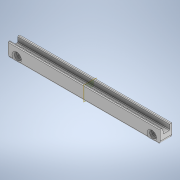
# Autodesk Inventor part: DisplayHolderLower
Saved by Autodesk Inventor 2022 (Build 260153000, 153)
## iProperties
Created: 2021-04-23
Part Number: DisplayHolderLower
Material: Generic
Document SubType Name: Modeling
Designer: Viktor
Density: 1 g/cm^3
Appearance: Default
Author: Viktor
## iProperties of the stored document DisplayHolderLower_3DPrint.ipt
Created: 2021-04-23
Part Number: DisplayHolderLower_3DPrint
Material: Generic
Document SubType Name: Modeling
Designer: Viktor
Density: 1 g/cm^3
Appearance: Default
Author: Viktor
Autodesk Inventor part; units mm, degrees
ref_plane "YZ Plane" through (0, 0, 0) normal (1, 0, 0) x (0, 1, 0)
ref_plane "XZ Plane" through (0, 0, 0) normal (0, 1, 0) x (-1, 0, 0)
ref_plane "XY Plane" through (0, 0, 0) normal (0, 0, 1) x (1, 0, 0)
sketch "Sketch1" plane through (0, 0, 0) normal (0, 0, 1) x (1, 0, 0)
  line L0 (-12.5, -10) -> (12.5, -10)
  line L1 (12.5, -10) -> (12.5, 10)
  line L2 (12.5, 10) -> (-12.5, 10)
  line L3 (-12.5, 10) -> (-12.5, -10)
  line L4 (-12.5, -10) -> (12.5, 10) construction
  line L5 (12.5, -10) -> (-12.5, 10) construction
  point P0 (0, 0)
  dimension "d0" = 25
  dimension "d1" = 20
  constraints: 12 end point, 2 midpoint, 2 parallel, 1 horizontal, 1 perpendicular
  measures "d0" distance of L1.end L2.end
  measures "d1" distance of L0.end L1.end
extrude "Extrusion1" add sketch "Sketch1" along normal blind 17
sketch "Sketch2" plane through (-12.5, 10, 0) normal (0, 1, 0) x (1, 0, 0)
  line L0 (0, 0) -> (0, -17) projected
  line L1 (25, 0) -> (25, -17) projected
  line L2 (0, -2.8) -> (25, -2.8)
  line L3 (25, -2.8) -> (25, -12.4)
  line L4 (25, -12.4) -> (0, -12.4)
  line L5 (0, -12.4) -> (0, -2.8)
  line L6 (25, 0) -> (0, 0) projected
  point P0 (12.5, 0)
  point P1 (0, -12.4)
  dimension "d4" = 2.8
  dimension "d5" = 9.6
  constraints: 8 end point, 2 parallel, 2 point on line, 1 horizontal, 1 perpendicular
  measures "d4" distance between parallel lines of L6 L2
  measures "d5" distance between parallel lines of L4 L2
extrude "Extrusion2" cut sketch "Sketch2" against normal blind 8 contours L2 L1 L4 L0
chamfer "Chamfer1" distance 2 angle 70 1 edges at (0, 10, 12.4) measured on face at (0, 10, 12.9)
fillet "Fillet1" radius 1 5 edges at (0, 2, 12.4) (0, 2, 2.8) (0, 10, 14.4) (0, 10, 17) (0, 10, 2.8)
sketch "Sketch3" plane through (0, 0, 17) normal (0, 0, 1) x (1, 0, 0)
  line L0 (0, 14) -> (0, -14) projected
  circle A0 centre (0, -4) radius 2.4
  line L1 (-12.5, -10) -> (12.5, -10) projected
  point P0 (0, 0)
  dimension "d12" = 4.8
  dimension "d13" = 6
  constraints: 1 centre point, 1 point on line
  measures "d12" diameter of A0
  measures "d13" distance from line of L1 A0.centre
extrude "Extrusion3" cut sketch "Sketch3" against normal through all
sketch "Sketch4" plane through (0, 0, 17) normal (0, 0, 1) x (1, 0, 0)
  circle A0 centre (0, -4) radius 2.4 projected
  circle A1 centre (0, -4) radius 5
  point P0 (0, 0)
  dimension "d16" = 10
  constraints: 1 centre point, 1 coincident
  measures "d16" diameter of A1
extrude "Extrusion4" cut sketch "Sketch4" against normal blind 5 contours A0 | A1
chamfer "Chamfer2" distance 2 angle 45 1 edges at (-5, -4, 17)
sketch "Sketch6" plane through (-12.5, -10, 0) normal (-1, 0, 0) x (0, 0, 1)
  arc A0 (2.8, 19) -> (1.8, 20) centre (1.8, 19) ccw projected
  line L0 (0, 20) -> (1.8, 20) projected
  line L1 (0, 20) -> (0, 0) projected
  line L2 (0, 0) -> (17, 0) projected
  line L3 (17, 19) -> (17, 0) projected
  arc A1 (17, 19) -> (16, 20) centre (16, 19) ccw projected
  line L4 (15.1002, 20) -> (16, 20) projected
  arc A2 (15.1002, 20) -> (14.1605, 19.342) centre (15.1002, 19) ccw projected
  line L5 (12.4, 14.505) -> (14.1605, 19.342) projected
  line L6 (12.4, 14.505) -> (12.4, 13) projected
  arc A3 (11.4, 12) -> (12.4, 13) centre (11.4, 13) ccw projected
  line L7 (11.4, 12) -> (3.8, 12) projected
  arc A4 (2.8, 13) -> (3.8, 12) centre (3.8, 13) ccw projected
  line L8 (2.8, 13) -> (2.8, 19) projected
  point P0 (0, 10)
extrude "Extrusion6" add sketch "Sketch6" along normal blind 87.5
ref_plane "Work Plane1" through (-100, -10, 0) normal (-1, 0, 0) x (0, 0, 1)
mirror "Mirror1" about plane through (-100, -10, 0) normal (-1, 0, 0) of "Extrusion1", "Extrusion2", "Chamfer1", "Fillet1", "Extrusion3", "Extrusion4", "Chamfer2", "Extrusion6"
fillet "Fillet3" radius 2 3 edges at (-100, -10, 17) (-208.0528, -10, 17) (8.0528, -10, 17)
fillet "Fillet3" radius 5 2 edges at (12.5, -10, 8.5) (-212.5, -10, 8.5)
body "Solid1"
